Autodesk Fusion 360 part; units mm, degrees
(part 3 of 3)
sketch "Sketch12" plane through (0, 0, 3) normal (0, 0, 1) x (-1, 0, 0)
  circle A0 centre (-5.4, -11) radius 2.5
  circle A1 centre (-5.4, -64) radius 2.5
  line L0 (-15, -66.5) -> (-15, -75)
  line L1 (-15, -75) -> (-2.5, -75)
  arc A2 (-2.5, -75) -> (0, -72.5) centre (-2.5, -72.5) ccw
  line L2 (0, -72.5) -> (0, -60)
  line L3 (0, -60) -> (-8.5, -60)
  arc A3 (-11, -57.5) -> (-8.5, -60) centre (-8.5, -57.5) ccw
  line L4 (-11, -57.5) -> (-11, -17.5)
  arc A4 (-8.5, -15) -> (-11, -17.5) centre (-8.5, -17.5) ccw
  line L5 (-8.5, -15) -> (0, -15)
  line L6 (0, -15) -> (0, -2.5)
  arc A5 (0, -2.5) -> (-2.5, 0) centre (-2.5, -2.5) ccw
  line L7 (-2.5, 0) -> (-57.5, 0)
  arc A6 (-57.5, 0) -> (-60, -2.5) centre (-57.5, -2.5) ccw
  line L8 (-60, -2.5) -> (-60, -25)
  line L9 (-60, -25) -> (-51.5, -25)
  arc A7 (-49, -27.5) -> (-51.5, -25) centre (-51.5, -27.5) ccw
  line L10 (-49, -27.5) -> (-49, -56.5)
  arc A8 (-51.5, -59) -> (-49, -56.5) centre (-51.5, -56.5) ccw
  line L11 (-51.5, -59) -> (-60, -59)
  line L12 (-60, -59) -> (-60, -72.5)
  arc A9 (-60, -72.5) -> (-57.5, -75) centre (-57.5, -72.5) ccw
  line L13 (-57.5, -75) -> (-45, -75)
  line L14 (-45, -75) -> (-45, -66.5)
  arc A10 (-42.5, -64) -> (-45, -66.5) centre (-42.5, -66.5) ccw
  line L15 (-42.5, -64) -> (-17.5, -64)
  arc A11 (-15, -66.5) -> (-17.5, -64) centre (-17.5, -66.5) ccw
  line L16 (-31.117, -41.7434) -> (-30.2084, -42.0729)
  line L17 (-30.2084, -42.0729) -> (-30.2084, -42.4945)
  line L18 (-30.2084, -42.4945) -> (-33.2084, -41.3423)
  line L19 (-33.2084, -41.3423) -> (-33.2084, -40.9146)
  line L20 (-33.2084, -40.9146) -> (-30.2084, -39.6868)
  line L21 (-30.2084, -39.6868) -> (-30.2084, -40.1391)
  line L22 (-30.2084, -40.1391) -> (-31.117, -40.489)
  line L23 (-31.117, -40.489) -> (-31.117, -41.7434)
  line L24 (-32.8544, -35.9604) -> (-30.2084, -35.9604)
  line L25 (-30.2084, -35.9604) -> (-30.2084, -36.3573)
  line L26 (-30.2084, -36.3573) -> (-32.8544, -36.3573)
  line L27 (-32.8544, -36.3573) -> (-32.8544, -37.3458)
  line L28 (-32.8544, -37.3458) -> (-33.2084, -37.3458)
  line L29 (-33.2084, -37.3458) -> (-33.2084, -34.9679)
  line L30 (-33.2084, -34.9679) -> (-32.8544, -34.9679)
  line L31 (-32.8544, -34.9679) -> (-32.8544, -35.9604)
  line L32 (-31.5406, -31.3621) -> (-30.2084, -31.3621)
  line L33 (-30.2084, -31.3621) -> (-30.2084, -31.7591)
  line L34 (-30.2084, -31.7591) -> (-33.2084, -31.7591)
  line L35 (-33.2084, -31.7591) -> (-33.2084, -30.429)
  spline S0 degree 3 poles (-33.2084, -30.429) (-33.2075, -30.3105) (-33.2059, -30.1035) (-33.151, -29.9043) (-33.1276, -29.8192) knots 0 0 0 0 0.035358 0.061746 0.061746 0.061746 0.061746
  spline S1 degree 3 poles (-33.1276, -29.8192) (-33.0949, -29.7527) (-33.0282, -29.6173) (-32.9049, -29.53) (-32.8421, -29.4856) knots 0 0 0 0 0.021851 0.044529 0.044529 0.044529 0.044529
  spline S2 degree 3 poles (-32.8421, -29.4856) (-32.7718, -29.4492) (-32.6298, -29.3757) (-32.4703, -29.3658) (-32.3899, -29.3608) knots 0 0 0 0 0.023485 0.047377 0.047377 0.047377 0.047377
  spline S3 degree 3 poles (-32.3899, -29.3608) (-32.2883, -29.3688) (-32.0883, -29.3846) (-31.9297, -29.5072) (-31.8517, -29.5674) knots 0 0 0 0 0.029867 0.058777 0.058777 0.058777 0.058777
  spline S4 degree 3 poles (-31.8517, -29.5674) (-31.7846, -29.6517) (-31.6358, -29.839) (-31.5955, -30.0758) (-31.5734, -30.2059) knots 0 0 0 0 0.031814 0.070654 0.070654 0.070654 0.070654
  spline S5 degree 3 poles (-31.5734, -30.2059) (-31.55, -30.1586) (-31.5081, -30.0738) (-31.4498, -29.9994) (-31.424, -29.9665) knots 0 0 0 0 0.015773 0.028287 0.028287 0.028287 0.028287
  spline S6 degree 3 poles (-31.424, -29.9665) (-31.3657, -29.9082) (-31.2433, -29.7856) (-31.1, -29.6881) (-31.0249, -29.637) knots 0 0 0 0 0.024682 0.05185 0.05185 0.05185 0.05185
  line L36 (-31.0249, -29.637) -> (-30.2084, -29.1152)
  line L37 (-30.2084, -29.1152) -> (-30.2084, -29.6145)
  line L38 (-30.2084, -29.6145) -> (-30.8326, -30.0115)
  spline S7 degree 3 poles (-30.8326, -30.0115) (-30.9127, -30.0634) (-31.0536, -30.1545) (-31.188, -30.2548) (-31.2459, -30.298) knots 0 0 0 0 0.028634 0.050307 0.050307 0.050307 0.050307
  spline S8 degree 3 poles (-31.2459, -30.298) (-31.2883, -30.3319) (-31.3628, -30.3915) (-31.4212, -30.467) (-31.4465, -30.4996) knots 0 0 0 0 0.016187 0.028522 0.028522 0.028522 0.028522
  spline S9 degree 3 poles (-31.4465, -30.4996) (-31.464, -30.5289) (-31.4981, -30.586) (-31.5171, -30.6497) (-31.5263, -30.6807) knots 0 0 0 0 0.010209 0.01986 0.01986 0.01986 0.01986
  spline S10 degree 3 poles (-31.5263, -30.6807) (-31.5304, -30.7103) (-31.5407, -30.7836) (-31.5406, -30.8576) (-31.5406, -30.9017) knots 0 0 0 0 0.008966 0.02217 0.02217 0.02217 0.02217
  line L39 (-31.5406, -30.9017) -> (-31.5406, -31.3621)
  line L40 (-31.4792, -27.5722) -> (-30.2084, -27.5722)
  line L41 (-30.2084, -27.5722) -> (-30.2084, -27.9692)
  line L42 (-30.2084, -27.9692) -> (-31.4792, -27.9692)
  line L43 (-31.4792, -27.9692) -> (-33.2084, -29.1254)
  line L44 (-33.2084, -29.1254) -> (-33.2084, -28.6425)
  line L45 (-33.2084, -28.6425) -> (-32.3039, -28.0511)
  spline S11 degree 3 poles (-32.3039, -28.0511) (-32.2198, -27.9977) (-32.0531, -27.8919) (-31.8814, -27.7944) (-31.7964, -27.7462) knots 0 0 0 0 0.029896 0.059213 0.059213 0.059213 0.059213
  spline S12 degree 3 poles (-31.7964, -27.7462) (-31.8801, -27.6969) (-32.0592, -27.5916) (-32.2336, -27.4788) (-32.3264, -27.4187) knots 0 0 0 0 0.029138 0.062305 0.062305 0.062305 0.062305
  line L46 (-32.3264, -27.4187) -> (-33.2084, -26.8376)
  line L47 (-33.2084, -26.8376) -> (-33.2084, -26.3751)
  line L48 (-33.2084, -26.3751) -> (-31.4792, -27.5722)
  line L49 (-31.117, -22.178) -> (-30.2084, -22.5074)
  line L50 (-30.2084, -22.5074) -> (-30.2084, -22.929)
  line L51 (-30.2084, -22.929) -> (-33.2084, -21.7769)
  line L52 (-33.2084, -21.7769) -> (-33.2084, -21.3492)
  line L53 (-33.2084, -21.3492) -> (-30.2084, -20.1213)
  line L54 (-30.2084, -20.1213) -> (-30.2084, -20.5736)
  line L55 (-30.2084, -20.5736) -> (-31.117, -20.9235)
  line L56 (-31.117, -20.9235) -> (-31.117, -22.178)
  line L57 (-30.5624, -15.0729) -> (-30.2084, -15.0729)
  line L58 (-30.2084, -15.0729) -> (-30.2084, -17.3116)
  line L59 (-30.2084, -17.3116) -> (-33.2084, -17.3116)
  line L60 (-33.2084, -17.3116) -> (-33.2084, -15.1425)
  line L61 (-33.2084, -15.1425) -> (-32.8544, -15.1425)
  line L62 (-32.8544, -15.1425) -> (-32.8544, -16.9147)
  line L63 (-32.8544, -16.9147) -> (-31.9356, -16.9147)
  line L64 (-31.9356, -16.9147) -> (-31.9356, -15.255)
  line L65 (-31.9356, -15.255) -> (-31.5836, -15.255)
  line L66 (-31.5836, -15.255) -> (-31.5836, -16.9147)
  line L67 (-31.5836, -16.9147) -> (-30.5624, -16.9147)
  line L68 (-30.5624, -16.9147) -> (-30.5624, -15.0729)
  line L69 (-31.4792, -18.873) -> (-30.2084, -18.873)
  line L70 (-30.2084, -18.873) -> (-30.2084, -19.27)
  line L71 (-30.2084, -19.27) -> (-31.4792, -19.27)
  line L72 (-31.4792, -19.27) -> (-33.2084, -20.4262)
  line L73 (-33.2084, -20.4262) -> (-33.2084, -19.9433)
  line L74 (-33.2084, -19.9433) -> (-32.3039, -19.3519)
  spline S13 degree 3 poles (-32.3039, -19.3519) (-32.2198, -19.2985) (-32.0531, -19.1927) (-31.8814, -19.0952) (-31.7964, -19.047) knots 0 0 0 0 0.029897 0.059214 0.059214 0.059214 0.059214
  spline S14 degree 3 poles (-31.7964, -19.047) (-31.8801, -18.9977) (-32.0592, -18.8924) (-32.2336, -18.7796) (-32.3264, -18.7196) knots 0 0 0 0 0.029138 0.062305 0.062305 0.062305 0.062305
  line L75 (-32.3264, -18.7196) -> (-33.2084, -18.1384)
  line L76 (-33.2084, -18.1384) -> (-33.2084, -17.6759)
  line L77 (-33.2084, -17.6759) -> (-31.4792, -18.873)
  line L78 (-30.5624, -23.0722) -> (-30.2084, -23.0722)
  line L79 (-30.2084, -23.0722) -> (-30.2084, -24.9467)
  line L80 (-30.2084, -24.9467) -> (-33.2084, -24.9467)
  line L81 (-33.2084, -24.9467) -> (-33.2084, -24.5497)
  line L82 (-33.2084, -24.5497) -> (-30.5624, -24.5497)
  line L83 (-30.5624, -24.5497) -> (-30.5624, -23.0722)
  line L84 (-31.5406, -14.1213) -> (-30.2084, -14.1213)
  line L85 (-30.2084, -14.1213) -> (-30.2084, -14.5183)
  line L86 (-30.2084, -14.5183) -> (-33.2084, -14.5183)
  line L87 (-33.2084, -14.5183) -> (-33.2084, -13.1882)
  spline S15 degree 3 poles (-33.2084, -13.1882) (-33.2075, -13.0697) (-33.2059, -12.8627) (-33.151, -12.6635) (-33.1276, -12.5784) knots 0 0 0 0 0.035358 0.061746 0.061746 0.061746 0.061746
  spline S16 degree 3 poles (-33.1276, -12.5784) (-33.0949, -12.5119) (-33.0282, -12.3765) (-32.9049, -12.2892) (-32.8421, -12.2448) knots 0 0 0 0 0.021851 0.044528 0.044528 0.044528 0.044528
  spline S17 degree 3 poles (-32.8421, -12.2448) (-32.7718, -12.2084) (-32.6298, -12.1349) (-32.4703, -12.125) (-32.3899, -12.12) knots 0 0 0 0 0.023485 0.047377 0.047377 0.047377 0.047377
  spline S18 degree 3 poles (-32.3899, -12.12) (-32.2883, -12.128) (-32.0883, -12.1438) (-31.9297, -12.2664) (-31.8517, -12.3267) knots 0 0 0 0 0.029867 0.058777 0.058777 0.058777 0.058777
  spline S19 degree 3 poles (-31.8517, -12.3267) (-31.7846, -12.411) (-31.6358, -12.5982) (-31.5955, -12.835) (-31.5734, -12.9651) knots 0 0 0 0 0.031814 0.070654 0.070654 0.070654 0.070654
  spline S20 degree 3 poles (-31.5734, -12.9651) (-31.55, -12.9178) (-31.5081, -12.833) (-31.4498, -12.7586) (-31.424, -12.7257) knots 0 0 0 0 0.015772 0.028287 0.028287 0.028287 0.028287
  spline S21 degree 3 poles (-31.424, -12.7257) (-31.3657, -12.6674) (-31.2433, -12.5448) (-31.1, -12.4473) (-31.0249, -12.3962) knots 0 0 0 0 0.024682 0.05185 0.05185 0.05185 0.05185
  line L88 (-31.0249, -12.3962) -> (-30.2084, -11.8744)
  line L89 (-30.2084, -11.8744) -> (-30.2084, -12.3737)
  line L90 (-30.2084, -12.3737) -> (-30.8326, -12.7707)
  spline S22 degree 3 poles (-30.8326, -12.7707) (-30.9127, -12.8226) (-31.0535, -12.9137) (-31.188, -13.014) (-31.2459, -13.0572) knots 0 0 0 0 0.028634 0.050306 0.050306 0.050306 0.050306
  spline S23 degree 3 poles (-31.2459, -13.0572) (-31.2883, -13.0911) (-31.3628, -13.1507) (-31.4212, -13.2262) (-31.4465, -13.2588) knots 0 0 0 0 0.016188 0.028522 0.028522 0.028522 0.028522
  spline S24 degree 3 poles (-31.4465, -13.2588) (-31.464, -13.2881) (-31.4981, -13.3452) (-31.5171, -13.4089) (-31.5263, -13.4399) knots 0 0 0 0 0.010209 0.01986 0.01986 0.01986 0.01986
  spline S25 degree 3 poles (-31.5263, -13.4399) (-31.5304, -13.4695) (-31.5407, -13.5428) (-31.5406, -13.6168) (-31.5406, -13.6609) knots 0 0 0 0 0.008967 0.02217 0.02217 0.02217 0.02217
  line L91 (-31.5406, -13.6609) -> (-31.5406, -14.1213)
  line L92 (-30.5624, -32.3137) -> (-30.2084, -32.3137)
  line L93 (-30.2084, -32.3137) -> (-30.2084, -34.5524)
  line L94 (-30.2084, -34.5524) -> (-33.2084, -34.5524)
  line L95 (-33.2084, -34.5524) -> (-33.2084, -32.3833)
  line L96 (-33.2084, -32.3833) -> (-32.8544, -32.3833)
  line L97 (-32.8544, -32.3833) -> (-32.8544, -34.1554)
  line L98 (-32.8544, -34.1554) -> (-31.9356, -34.1554)
  line L99 (-31.9356, -34.1554) -> (-31.9356, -32.4958)
  line L100 (-31.9356, -32.4958) -> (-31.5836, -32.4958)
  line L101 (-31.5836, -32.4958) -> (-31.5836, -34.1554)
  line L102 (-31.5836, -34.1554) -> (-30.5624, -34.1554)
  line L103 (-30.5624, -34.1554) -> (-30.5624, -32.3137)
  line L104 (-32.8544, -38.5204) -> (-30.2084, -38.5204)
  line L105 (-30.2084, -38.5204) -> (-30.2084, -38.9174)
  line L106 (-30.2084, -38.9174) -> (-32.8544, -38.9174)
  line L107 (-32.8544, -38.9174) -> (-32.8544, -39.9058)
  line L108 (-32.8544, -39.9058) -> (-33.2084, -39.9058)
  line L109 (-33.2084, -39.9058) -> (-33.2084, -37.5279)
  line L110 (-33.2084, -37.5279) -> (-32.8544, -37.5279)
  line L111 (-32.8544, -37.5279) -> (-32.8544, -38.5204)
  spline S26 degree 3 poles (-30.2586, -43.3488) (-30.244, -43.4218) (-30.212, -43.5815) (-30.2097, -43.7444) (-30.2084, -43.8328) knots 0 0 0 0 0.022292 0.048746 0.048746 0.048746 0.048746
  line L112 (-30.2084, -43.8328) -> (-30.2084, -44.9767)
  line L113 (-30.2084, -44.9767) -> (-33.2084, -44.9767)
  line L114 (-33.2084, -44.9767) -> (-33.2084, -43.8512)
  spline S27 degree 3 poles (-33.2084, -43.8512) (-33.2065, -43.747) (-33.2031, -43.5584) (-33.1438, -43.3796) (-33.1174, -43.2997) knots 0 0 0 0 0.031061 0.05618 0.05618 0.05618 0.05618
  spline S28 degree 3 poles (-33.1174, -43.2997) (-33.0831, -43.2343) (-33.0148, -43.1041) (-32.8961, -43.0175) (-32.837, -42.9743) knots 0 0 0 0 0.021833 0.043463 0.043463 0.043463 0.043463
  spline S29 degree 3 poles (-32.837, -42.9743) (-32.7739, -42.94) (-32.6502, -42.8727) (-32.5098, -42.862) (-32.441, -42.8567) knots 0 0 0 0 0.02128 0.041726 0.041726 0.041726 0.041726
  spline S30 degree 3 poles (-32.441, -42.8567) (-32.3776, -42.8612) (-32.2495, -42.8703) (-32.1361, -42.9306) (-32.0788, -42.961) knots 0 0 0 0 0.018855 0.038069 0.038069 0.038069 0.038069
  spline S31 degree 3 poles (-32.0788, -42.961) (-32.0242, -43.0017) (-31.9101, -43.0867) (-31.8408, -43.2112) (-31.8046, -43.2762) knots 0 0 0 0 0.020176 0.042199 0.042199 0.042199 0.042199
  spline S32 degree 3 poles (-31.8046, -43.2762) (-31.7748, -43.1919) (-31.7176, -43.0302) (-31.5924, -42.9135) (-31.5324, -42.8577) knots 0 0 0 0 0.02638 0.050582 0.050582 0.050582 0.050582
  spline S33 degree 3 poles (-31.5324, -42.8577) (-31.4645, -42.815) (-31.3256, -42.7278) (-31.1618, -42.7169) (-31.0781, -42.7114) knots 0 0 0 0 0.023673 0.048399 0.048399 0.048399 0.048399
  spline S34 degree 3 poles (-31.0781, -42.7114) (-31.0095, -42.7149) (-30.8737, -42.7219) (-30.7482, -42.7744) (-30.6863, -42.8004) knots 0 0 0 0 0.020457 0.040457 0.040457 0.040457 0.040457
  spline S35 degree 3 poles (-30.6863, -42.8004) (-30.6304, -42.8305) (-30.5243, -42.8876) (-30.4446, -42.9778) (-30.4069, -43.0204) knots 0 0 0 0 0.018875 0.035805 0.035805 0.035805 0.035805
  spline S36 degree 3 poles (-30.4069, -43.0204) (-30.3758, -43.0685) (-30.3098, -43.1704) (-30.2763, -43.2872) (-30.2586, -43.3488) knots 0 0 0 0 0.017093 0.036216 0.036216 0.036216 0.036216
  circle A12 centre (-54.6, -16.4) radius 1.4
  circle A13 centre (-5.4, -69.6) radius 1.4
  circle A14 centre (-5.4, -5.4) radius 1.4
  circle A15 centre (-54.6, -69.6) radius 1.4
  spline S37 degree 3 poles (-39.691, -3.4945) (-39.6372, -3.3999) (-39.5038, -3.1654) (-39.5044, -2.8934) (-39.5048, -2.7312) knots 0 0 0 0 0.032195 0.079746 0.079746 0.079746 0.079746
  line L115 (-39.5048, -2.7312) -> (-39.5048, -1)
  line L116 (-39.5048, -1) -> (-39.1078, -1)
  line L117 (-39.1078, -1) -> (-39.1078, -2.7333)
  spline S38 degree 3 poles (-39.1078, -2.7333) (-39.1097, -2.8695) (-39.1131, -3.1137) (-39.1804, -3.348) (-39.2101, -3.4516) knots 0 0 0 0 0.04065 0.072837 0.072837 0.072837 0.072837
  spline S39 degree 3 poles (-39.2101, -3.4516) (-39.2522, -3.5368) (-39.3388, -3.712) (-39.4978, -3.8259) (-39.5795, -3.8844) knots 0 0 0 0 0.028068 0.057686 0.057686 0.057686 0.057686
  spline S40 degree 3 poles (-39.5795, -3.8844) (-39.6807, -3.9329) (-39.9017, -4.039) (-40.1472, -4.0469) (-40.2804, -4.0512) knots 0 0 0 0 0.033312 0.072747 0.072747 0.072747 0.072747
  spline S41 degree 3 poles (-40.2804, -4.0512) (-40.4099, -4.0474) (-40.649, -4.0405) (-40.8692, -3.9482) (-40.97, -3.9059) knots 0 0 0 0 0.03849 0.071015 0.071015 0.071015 0.071015
  spline S42 degree 3 poles (-40.97, -3.9059) (-41.0528, -3.8523) (-41.2175, -3.7458) (-41.3078, -3.5718) (-41.3527, -3.4853) knots 0 0 0 0 0.029047 0.057739 0.057739 0.057739 0.057739
  spline S43 degree 3 poles (-41.3527, -3.4853) (-41.386, -3.3776) (-41.4615, -3.133) (-41.4652, -2.8767) (-41.4673, -2.7333) knots 0 0 0 0 0.033678 0.076416 0.076416 0.076416 0.076416
  line L118 (-41.4673, -2.7333) -> (-41.4673, -1)
  line L119 (-41.4673, -1) -> (-41.0703, -1)
  line L120 (-41.0703, -1) -> (-41.0703, -2.7312)
  spline S44 degree 3 poles (-41.0703, -2.7312) (-41.0699, -2.8452) (-41.0692, -3.0405) (-41.0187, -3.2288) (-40.9976, -3.3073) knots 0 0 0 0 0.033993 0.058274 0.058274 0.058274 0.058274
  spline S45 degree 3 poles (-40.9976, -3.3073) (-40.9689, -3.3656) (-40.911, -3.4829) (-40.8025, -3.556) (-40.748, -3.5928) knots 0 0 0 0 0.01914 0.038515 0.038515 0.038515 0.038515
  spline S46 degree 3 poles (-40.748, -3.5928) (-40.6834, -3.622) (-40.546, -3.6841) (-40.3951, -3.69) (-40.3151, -3.693) knots 0 0 0 0 0.021059 0.044802 0.044802 0.044802 0.044802
  spline S47 degree 3 poles (-40.3151, -3.693) (-40.1854, -3.6901) (-39.9561, -3.685) (-39.7713, -3.5522) (-39.691, -3.4945) knots 0 0 0 0 0.037827 0.066851 0.066851 0.066851 0.066851
  spline S48 degree 3 poles (-34.0399, -3.9499) (-34.1129, -3.9645) (-34.2726, -3.9964) (-34.4355, -3.9987) (-34.5239, -4) knots 0 0 0 0 0.022292 0.048746 0.048746 0.048746 0.048746
  line L121 (-34.5239, -4) -> (-35.6678, -4)
  line L122 (-35.6678, -4) -> (-35.6678, -1)
  line L123 (-35.6678, -1) -> (-34.5423, -1)
  spline S49 degree 3 poles (-34.5423, -1) (-34.438, -1.0019) (-34.2495, -1.0053) (-34.0707, -1.0646) (-33.9908, -1.0911) knots 0 0 0 0 0.031061 0.05618 0.05618 0.05618 0.05618
  spline S50 degree 3 poles (-33.9908, -1.0911) (-33.9254, -1.1254) (-33.7952, -1.1936) (-33.7085, -1.3123) (-33.6654, -1.3714) knots 0 0 0 0 0.021833 0.043463 0.043463 0.043463 0.043463
  spline S51 degree 3 poles (-33.6654, -1.3714) (-33.6311, -1.4345) (-33.5638, -1.5583) (-33.553, -1.6986) (-33.5477, -1.7674) knots 0 0 0 0 0.02128 0.041726 0.041726 0.041726 0.041726
  spline S52 degree 3 poles (-33.5477, -1.7674) (-33.5523, -1.8308) (-33.5614, -1.9589) (-33.6217, -2.0724) (-33.6521, -2.1296) knots 0 0 0 0 0.018855 0.038069 0.038069 0.038069 0.038069
  spline S53 degree 3 poles (-33.6521, -2.1296) (-33.6928, -2.1842) (-33.7778, -2.2983) (-33.9023, -2.3676) (-33.9673, -2.4038) knots 0 0 0 0 0.020176 0.042199 0.042199 0.042199 0.042199
  spline S54 degree 3 poles (-33.9673, -2.4038) (-33.8829, -2.4336) (-33.7213, -2.4908) (-33.6046, -2.6161) (-33.5488, -2.676) knots 0 0 0 0 0.02638 0.050582 0.050582 0.050582 0.050582
  spline S55 degree 3 poles (-33.5488, -2.676) (-33.5061, -2.7439) (-33.4189, -2.8828) (-33.408, -3.0466) (-33.4025, -3.1303) knots 0 0 0 0 0.023673 0.048399 0.048399 0.048399 0.048399
  spline S56 degree 3 poles (-33.4025, -3.1303) (-33.406, -3.199) (-33.413, -3.3348) (-33.4655, -3.4602) (-33.4915, -3.5222) knots 0 0 0 0 0.020457 0.040457 0.040457 0.040457 0.040457
  spline S57 degree 3 poles (-33.4915, -3.5222) (-33.5216, -3.5781) (-33.5787, -3.6841) (-33.6688, -3.7638) (-33.7115, -3.8015) knots 0 0 0 0 0.018874 0.035805 0.035805 0.035805 0.035805
  spline S58 degree 3 poles (-33.7115, -3.8015) (-33.7596, -3.8326) (-33.8615, -3.8986) (-33.9782, -3.9322) (-34.0399, -3.9499) knots 0 0 0 0 0.017093 0.036216 0.036216 0.036216 0.036216
  line L124 (-31.2947, -2.7804) -> (-31.2947, -4)
  line L125 (-31.2947, -4) -> (-31.6917, -4)
  line L126 (-31.6917, -4) -> (-31.6917, -1)
  line L127 (-31.6917, -1) -> (-30.56, -1)
  spline S59 degree 3 poles (-30.56, -1) (-30.4721, -1.0003) (-30.3193, -1.0007) (-30.1679, -1.0203) (-30.1037, -1.0286) knots 0 0 0 0 0.026357 0.045763 0.045763 0.045763 0.045763
  spline S60 degree 3 poles (-30.1037, -1.0286) (-30.0345, -1.0427) (-29.9033, -1.0693) (-29.7879, -1.1369) (-29.7333, -1.1688) knots 0 0 0 0 0.021002 0.039845 0.039845 0.039845 0.039845
  spline S61 degree 3 poles (-29.7333, -1.1688) (-29.6854, -1.2077) (-29.5863, -1.2884) (-29.5247, -1.4004) (-29.4928, -1.4584) knots 0 0 0 0 0.01832 0.037955 0.037955 0.037955 0.037955
  spline S62 degree 3 poles (-29.4928, -1.4584) (-29.4663, -1.5227) (-29.4121, -1.6538) (-29.4053, -1.7955) (-29.4018, -1.8677) knots 0 0 0 0 0.020702 0.042208 0.042208 0.042208 0.042208
  spline S63 degree 3 poles (-29.4018, -1.8677) (-29.4112, -1.9895) (-29.4298, -2.2292) (-29.5743, -2.4211) (-29.6453, -2.5153) knots 0 0 0 0 0.035846 0.070494 0.070494 0.070494 0.070494
  spline S64 degree 3 poles (-29.6453, -2.5153) (-29.7556, -2.5922) (-30.0174, -2.7744) (-30.3391, -2.7782) (-30.5252, -2.7804) knots 0 0 0 0 0.039534 0.09376 0.09376 0.09376 0.09376
  line L128 (-30.5252, -2.7804) -> (-31.2947, -2.7804)
  line L129 (-25.2333, -2.6678) -> (-25.2333, -4)
  line L130 (-25.2333, -4) -> (-25.6303, -4)
  line L131 (-25.6303, -4) -> (-25.6303, -1)
  line L132 (-25.6303, -1) -> (-24.3001, -1)
  spline S65 degree 3 poles (-24.3001, -1) (-24.1816, -1.0009) (-23.9747, -1.0025) (-23.7754, -1.0574) (-23.6903, -1.0808) knots 0 0 0 0 0.035358 0.061746 0.061746 0.061746 0.061746
  spline S66 degree 3 poles (-23.6903, -1.0808) (-23.6239, -1.1135) (-23.4884, -1.1802) (-23.4012, -1.3035) (-23.3568, -1.3663) knots 0 0 0 0 0.021851 0.044529 0.044529 0.044529 0.044529
  spline S67 degree 3 poles (-23.3568, -1.3663) (-23.3203, -1.4367) (-23.2469, -1.5786) (-23.2369, -1.7381) (-23.2319, -1.8186) knots 0 0 0 0 0.023485 0.047377 0.047377 0.047377 0.047377
  spline S68 degree 3 poles (-23.2319, -1.8186) (-23.24, -1.9202) (-23.2558, -2.1202) (-23.3783, -2.2787) (-23.4386, -2.3568) knots 0 0 0 0 0.029867 0.058777 0.058777 0.058777 0.058777
  spline S69 degree 3 poles (-23.4386, -2.3568) (-23.5229, -2.4238) (-23.7101, -2.5726) (-23.9469, -2.6129) (-24.0771, -2.6351) knots 0 0 0 0 0.031814 0.070654 0.070654 0.070654 0.070654
  spline S70 degree 3 poles (-24.0771, -2.6351) (-24.0298, -2.6584) (-23.945, -2.7003) (-23.8706, -2.7587) (-23.8377, -2.7844) knots 0 0 0 0 0.015773 0.028287 0.028287 0.028287 0.028287
  spline S71 degree 3 poles (-23.8377, -2.7844) (-23.7793, -2.8427) (-23.6568, -2.9652) (-23.5593, -3.1084) (-23.5082, -3.1835) knots 0 0 0 0 0.024682 0.05185 0.05185 0.05185 0.05185
  line L133 (-23.5082, -3.1835) -> (-22.9864, -4)
  line L134 (-22.9864, -4) -> (-23.4857, -4)
  line L135 (-23.4857, -4) -> (-23.8827, -3.3759)
  spline S72 degree 3 poles (-23.8827, -3.3759) (-23.9346, -3.2957) (-24.0257, -3.1549) (-24.126, -3.0204) (-24.1692, -2.9625) knots 0 0 0 0 0.028634 0.050307 0.050307 0.050307 0.050307
  spline S73 degree 3 poles (-24.1692, -2.9625) (-24.203, -2.9202) (-24.2627, -2.8456) (-24.3381, -2.7872) (-24.3707, -2.7619) knots 0 0 0 0 0.016188 0.028522 0.028522 0.028522 0.028522
  spline S74 degree 3 poles (-24.3707, -2.7619) (-24.4001, -2.7444) (-24.4572, -2.7103) (-24.5209, -2.6913) (-24.5518, -2.6821) knots 0 0 0 0 0.01021 0.01986 0.01986 0.01986 0.01986
  spline S75 degree 3 poles (-24.5518, -2.6821) (-24.5815, -2.678) (-24.6547, -2.6677) (-24.7288, -2.6678) (-24.7728, -2.6678) knots 0 0 0 0 0.008966 0.02217 0.02217 0.02217 0.02217
  line L136 (-24.7728, -2.6678) -> (-25.2333, -2.6678)
  spline S76 degree 3 poles (-28.3397, -3.8465) (-28.4442, -3.772) (-28.6535, -3.6227) (-28.7812, -3.3996) (-28.8452, -3.2879) knots 0 0 0 0 0.038012 0.076138 0.076138 0.076138 0.076138
  spline S77 degree 3 poles (-28.8452, -3.2879) (-28.8953, -3.1681) (-28.9957, -2.9283) (-29.0099, -2.6688) (-29.0171, -2.5389) knots 0 0 0 0 0.03864 0.077351 0.077351 0.077351 0.077351
  spline S78 degree 3 poles (-29.0171, -2.5389) (-29.0054, -2.3091) (-28.9837, -1.8792) (-28.7328, -1.5313) (-28.616, -1.3694) knots 0 0 0 0 0.067335 0.126001 0.126001 0.126001 0.126001
  spline S79 degree 3 poles (-28.616, -1.3694) (-28.4701, -1.2461) (-28.1712, -0.9936) (-27.7805, -0.9626) (-27.5805, -0.9468) knots 0 0 0 0 0.055813 0.114379 0.114379 0.114379 0.114379
  spline S80 degree 3 poles (-27.5805, -0.9468) (-27.4465, -0.9545) (-27.1831, -0.9695) (-26.9473, -1.0874) (-26.8315, -1.1453) knots 0 0 0 0 0.039806 0.078211 0.078211 0.078211 0.078211
  spline S81 degree 3 poles (-26.8315, -1.1453) (-26.7268, -1.2183) (-26.5162, -1.365) (-26.3876, -1.5872) (-26.323, -1.6988) knots 0 0 0 0 0.037796 0.075988 0.075988 0.075988 0.075988
  spline S82 degree 3 poles (-26.323, -1.6988) (-26.272, -1.8235) (-26.1664, -2.0815) (-26.1543, -2.3601) (-26.148, -2.5041) knots 0 0 0 0 0.040092 0.082957 0.082957 0.082957 0.082957
  spline S83 degree 3 poles (-26.148, -2.5041) (-26.1547, -2.6502) (-26.1676, -2.9335) (-26.2785, -3.1943) (-26.3322, -3.3206) knots 0 0 0 0 0.043474 0.084303 0.084303 0.084303 0.084303
  spline S84 degree 3 poles (-26.3322, -3.3206) (-26.3992, -3.4329) (-26.5315, -3.6547) (-26.7475, -3.7962) (-26.854, -3.866) knots 0 0 0 0 0.038684 0.076365 0.076365 0.076365 0.076365
  spline S85 degree 3 poles (-26.854, -3.866) (-26.969, -3.92) (-27.2, -4.0284) (-27.4547, -4.0436) (-27.5825, -4.0512) knots 0 0 0 0 0.037744 0.075783 0.075783 0.075783 0.075783
  spline S86 degree 3 poles (-27.5825, -4.0512) (-27.7188, -4.0434) (-27.9856, -4.0281) (-28.2233, -3.9062) (-28.3397, -3.8465) knots 0 0 0 0 0.040434 0.079208 0.079208 0.079208 0.079208
  line L137 (-21.5252, -1.354) -> (-21.5252, -4)
  line L138 (-21.5252, -4) -> (-21.9222, -4)
  line L139 (-21.9222, -4) -> (-21.9222, -1.354)
  line L140 (-21.9222, -1.354) -> (-22.9106, -1.354)
  line L141 (-22.9106, -1.354) -> (-22.9106, -1)
  line L142 (-22.9106, -1) -> (-20.5327, -1)
  line L143 (-20.5327, -1) -> (-20.5327, -1.354)
  line L144 (-20.5327, -1.354) -> (-21.5252, -1.354)
  spline S87 degree 3 poles (-37.9853, -3.9325) (-38.0718, -3.8885) (-38.2424, -3.8016) (-38.3594, -3.6501) (-38.4171, -3.5754) knots 0 0 0 0 0.028704 0.056657 0.056657 0.056657 0.056657
  spline S88 degree 3 poles (-38.4171, -3.5754) (-38.4631, -3.4926) (-38.5565, -3.3247) (-38.5733, -3.1332) (-38.5819, -3.0362) knots 0 0 0 0 0.02807 0.056948 0.056948 0.056948 0.056948
  line L145 (-38.5819, -3.0362) -> (-38.2074, -3.0034)
  spline S89 degree 3 poles (-38.2074, -3.0034) (-38.1968, -3.0732) (-38.177, -3.2037) (-38.1133, -3.3191) (-38.0836, -3.3728) knots 0 0 0 0 0.020962 0.039233 0.039233 0.039233 0.039233
  spline S90 degree 3 poles (-38.0836, -3.3728) (-38.0447, -3.4194) (-37.9614, -3.5192) (-37.8442, -3.5759) (-37.7817, -3.6061) knots 0 0 0 0 0.018003 0.038541 0.038541 0.038541 0.038541
  spline S91 degree 3 poles (-37.7817, -3.6061) (-37.71, -3.632) (-37.5612, -3.6858) (-37.4031, -3.6919) (-37.3213, -3.6951) knots 0 0 0 0 0.022745 0.047147 0.047147 0.047147 0.047147
  spline S92 degree 3 poles (-37.3213, -3.6951) (-37.2494, -3.6929) (-37.1125, -3.6887) (-36.9821, -3.6472) (-36.9202, -3.6276) knots 0 0 0 0 0.021451 0.040849 0.040849 0.040849 0.040849
  spline S93 degree 3 poles (-36.9202, -3.6276) (-36.867, -3.6044) (-36.7673, -3.5611) (-36.6951, -3.4801) (-36.6613, -3.4424) knots 0 0 0 0 0.017152 0.032166 0.032166 0.032166 0.032166
  spline S94 degree 3 poles (-36.6613, -3.4424) (-36.6366, -3.4025) (-36.5876, -3.3237) (-36.5801, -3.2312) (-36.5764, -3.1855) knots 0 0 0 0 0.013855 0.0274 0.0274 0.0274 0.0274
  spline S95 degree 3 poles (-36.5764, -3.1855) (-36.5796, -3.1402) (-36.5859, -3.051) (-36.6344, -2.9759) (-36.6583, -2.9389) knots 0 0 0 0 0.013382 0.02636 0.02636 0.02636 0.02636
  spline S96 degree 3 poles (-36.6583, -2.9389) (-36.6928, -2.9042) (-36.7701, -2.8264) (-36.872, -2.7849) (-36.9284, -2.7619) knots 0 0 0 0 0.014547 0.032588 0.032588 0.032588 0.032588
  spline S97 degree 3 poles (-36.9284, -2.7619) (-36.9928, -2.7413) (-37.1687, -2.6849) (-37.3486, -2.6425) (-37.4625, -2.6156) knots 0 0 0 0 0.0203 0.055396 0.055396 0.055396 0.055396
  spline S98 degree 3 poles (-37.4625, -2.6156) (-37.5809, -2.5873) (-37.779, -2.54) (-37.9663, -2.4604) (-38.0416, -2.4284) knots 0 0 0 0 0.036446 0.060956 0.060956 0.060956 0.060956
  spline S99 degree 3 poles (-38.0416, -2.4284) (-38.1076, -2.3903) (-38.2327, -2.318) (-38.3204, -2.2033) (-38.3619, -2.149) knots 0 0 0 0 0.022596 0.04287 0.04287 0.04287 0.04287
  spline S100 degree 3 poles (-38.3619, -2.149) (-38.3926, -2.0914) (-38.4548, -1.9746) (-38.4631, -1.8425) (-38.4673, -1.7756) knots 0 0 0 0 0.019362 0.039209 0.039209 0.039209 0.039209
  spline S101 degree 3 poles (-38.4673, -1.7756) (-38.4617, -1.7008) (-38.4504, -1.5497) (-38.3759, -1.4176) (-38.3383, -1.351) knots 0 0 0 0 0.022208 0.044864 0.044864 0.044864 0.044864
  spline S102 degree 3 poles (-38.3383, -1.351) (-38.2891, -1.2886) (-38.1871, -1.1594) (-38.0386, -1.088) (-37.9618, -1.0512) knots 0 0 0 0 0.02352 0.0487 0.0487 0.0487 0.0487
  spline S103 degree 3 poles (-37.9618, -1.0512) (-37.8755, -1.0213) (-37.6972, -0.9597) (-37.5086, -0.9525) (-37.4113, -0.9488) knots 0 0 0 0 0.027246 0.056264 0.056264 0.056264 0.056264
  spline S104 degree 3 poles (-37.4113, -0.9488) (-37.3057, -0.9524) (-37.1041, -0.9592) (-36.9136, -1.025) (-36.823, -1.0563) knots 0 0 0 0 0.031501 0.060107 0.060107 0.060107 0.060107
  spline S105 degree 3 poles (-36.823, -1.0563) (-36.7436, -1.0953) (-36.5891, -1.1713) (-36.4828, -1.3066) (-36.4311, -1.3724) knots 0 0 0 0 0.026156 0.050928 0.050928 0.050928 0.050928
  spline S106 degree 3 poles (-36.4311, -1.3724) (-36.3907, -1.445) (-36.3086, -1.5922) (-36.2921, -1.76) (-36.2838, -1.8452) knots 0 0 0 0 0.024624 0.04999 0.04999 0.04999 0.04999
  line L146 (-36.2838, -1.8452) -> (-36.6644, -1.8738)
  spline S107 degree 3 poles (-36.6644, -1.8738) (-36.6787, -1.7865) (-36.7056, -1.6222) (-36.819, -1.5009) (-36.8721, -1.4441) knots 0 0 0 0 0.025856 0.048693 0.048693 0.048693 0.048693
  spline S108 degree 3 poles (-36.8721, -1.4441) (-36.9434, -1.4018) (-37.1038, -1.3068) (-37.291, -1.3016) (-37.395, -1.2988) knots 0 0 0 0 0.024481 0.055061 0.055061 0.055061 0.055061
  spline S109 degree 3 poles (-37.395, -1.2988) (-37.5013, -1.3004) (-37.6877, -1.3032) (-37.8501, -1.3925) (-37.9198, -1.4308) knots 0 0 0 0 0.031305 0.054847 0.054847 0.054847 0.054847
  spline S110 degree 3 poles (-37.9198, -1.4308) (-37.9679, -1.4758) (-38.0606, -1.5627) (-38.0768, -1.6884) (-38.0846, -1.749) knots 0 0 0 0 0.019092 0.036842 0.036842 0.036842 0.036842
  spline S111 degree 3 poles (-38.0846, -1.749) (-38.0799, -1.8003) (-38.0706, -1.902) (-38.002, -1.9776) (-37.9679, -2.015) knots 0 0 0 0 0.01502 0.029764 0.029764 0.029764 0.029764
  spline S112 degree 3 poles (-37.9679, -2.015) (-37.9, -2.0529) (-37.7132, -2.157) (-37.5031, -2.2009) (-37.3694, -2.2289) knots 0 0 0 0 0.023235 0.063865 0.063865 0.063865 0.063865
  spline S113 degree 3 poles (-37.3694, -2.2289) (-37.2323, -2.2595) (-37.0069, -2.3098) (-36.7902, -2.3891) (-36.7053, -2.4202) knots 0 0 0 0 0.042069 0.06917 0.06917 0.06917 0.06917
  spline S114 degree 3 poles (-36.7053, -2.4202) (-36.6254, -2.4608) (-36.4756, -2.5368) (-36.3685, -2.6659) (-36.3186, -2.7261) knots 0 0 0 0 0.026563 0.04978 0.04978 0.04978 0.04978
  spline S115 degree 3 poles (-36.3186, -2.7261) (-36.2821, -2.791) (-36.2078, -2.9235) (-36.1985, -3.0753) (-36.1937, -3.1528) knots 0 0 0 0 0.022016 0.04497 0.04497 0.04497 0.04497
  spline S116 degree 3 poles (-36.1937, -3.1528) (-36.1997, -3.2319) (-36.212, -3.3924) (-36.2908, -3.5328) (-36.3308, -3.604) knots 0 0 0 0 0.023503 0.047671 0.047671 0.047671 0.047671
  spline S117 degree 3 poles (-36.3308, -3.604) (-36.3827, -3.6712) (-36.4898, -3.8099) (-36.6449, -3.8915) (-36.7248, -3.9335) knots 0 0 0 0 0.025169 0.051893 0.051893 0.051893 0.051893
  spline S118 degree 3 poles (-36.7248, -3.9335) (-36.8147, -3.9678) (-37.0008, -4.0388) (-37.2, -4.0469) (-37.3029, -4.0512) knots 0 0 0 0 0.028685 0.059343 0.059343 0.059343 0.059343
  spline S119 degree 3 poles (-37.3029, -4.0512) (-37.4288, -4.048) (-37.6624, -4.042) (-37.8835, -3.967) (-37.9853, -3.9325) knots 0 0 0 0 0.037541 0.069624 0.069624 0.069624 0.069624
  circle A16 centre (-54.6, -64) radius 2.5
  circle A17 centre (-54.6, -22) radius 2.5
  circle A18 centre (-5.4, -69.6) radius 2.75
  circle A19 centre (-54.6, -69.6) radius 2.75
  circle A20 centre (-54.6, -16.4) radius 2.75
  circle A21 centre (-5.4, -5.4) radius 2.75
  dimension "d89" = 5.5
  dimension "d90" = 5.5
  dimension "d91" = 5.5
  dimension "d92" = 5.5
  constraint concentric A13 A18
  constraint concentric A15 A19
  constraint concentric A12 A20
  constraint concentric A14 A21
  measures "d89" diameter of A18
  measures "d90" diameter of A19
  measures "d91" diameter of A20
  measures "d92" diameter of A21
extrude "Extrude13" cut sketch "Sketch12" against normal blind 1.5 contours A18
extrude "Extrude14" cut sketch "Sketch12" against normal blind 1.5 contours A19 | A20 | A21
sketch "Sketch13" plane through (0, 0, 0) normal (0, 0, -1) x (1, 0, 0)
  circle A0 centre (54.6, -69.6) radius 1.4
  circle A1 centre (5.4, -5.4) radius 1.4
  circle A2 centre (5.4, -69.6) radius 1.4
  circle A3 centre (54.6, -16.4) radius 1.4
  line L0 (15, -75) -> (15, -66.5)
  arc A4 (17.5, -64) -> (15, -66.5) centre (17.5, -66.5) ccw
  line L1 (17.5, -64) -> (42.5, -64)
  arc A5 (45, -66.5) -> (42.5, -64) centre (42.5, -66.5) ccw
  line L2 (45, -66.5) -> (45, -75)
  line L3 (45, -75) -> (57.5, -75)
  arc A6 (57.5, -75) -> (60, -72.5) centre (57.5, -72.5) ccw
  line L4 (60, -72.5) -> (60, -59)
  line L5 (60, -59) -> (51.5, -59)
  arc A7 (49, -56.5) -> (51.5, -59) centre (51.5, -56.5) ccw
  line L6 (49, -56.5) -> (49, -27.5)
  arc A8 (51.5, -25) -> (49, -27.5) centre (51.5, -27.5) ccw
  line L7 (51.5, -25) -> (60, -25)
  line L8 (60, -25) -> (60, -2.5)
  arc A9 (60, -2.5) -> (57.5, 0) centre (57.5, -2.5) ccw
  line L9 (57.5, 0) -> (2.5, 0)
  arc A10 (2.5, 0) -> (0, -2.5) centre (2.5, -2.5) ccw
  line L10 (0, -2.5) -> (0, -15)
  line L11 (0, -15) -> (8.5, -15)
  arc A11 (11, -17.5) -> (8.5, -15) centre (8.5, -17.5) ccw
  line L12 (11, -17.5) -> (11, -57.5)
  arc A12 (8.5, -60) -> (11, -57.5) centre (8.5, -57.5) ccw
  line L13 (8.5, -60) -> (0, -60)
  line L14 (0, -60) -> (0, -72.5)
  arc A13 (0, -72.5) -> (2.5, -75) centre (2.5, -72.5) ccw
  line L15 (2.5, -75) -> (15, -75)
  circle A14 centre (5.4, -11) radius 1.4
  circle A15 centre (54.6, -64) radius 1.4
  circle A16 centre (54.6, -22) radius 1.4
  circle A17 centre (5.4, -64) radius 1.4
  line L16 (56.0874, -24.8707) -> (57.8298, -22.1473)
  line L17 (57.8298, -22.1473) -> (56.3424, -19.2765)
  line L18 (56.3424, -19.2765) -> (53.1126, -19.1293)
  line L19 (53.1126, -19.1293) -> (51.3702, -21.8527)
  line L20 (51.3702, -21.8527) -> (52.8576, -24.7235)
  line L21 (52.8576, -24.7235) -> (56.0874, -24.8707)
  line L22 (52.1049, -61.9438) -> (51.5718, -65.1327)
  line L23 (51.5718, -65.1327) -> (54.0669, -67.1889)
  line L24 (54.0669, -67.1889) -> (57.0951, -66.0562)
  line L25 (57.0951, -66.0562) -> (57.6282, -62.8673)
  line L26 (57.6282, -62.8673) -> (55.1331, -60.8111)
  line L27 (55.1331, -60.8111) -> (52.1049, -61.9438)
  line L28 (7.2988, -61.3832) -> (4.0832, -61.0472)
  line L29 (4.0832, -61.0472) -> (2.1843, -63.664)
  line L30 (2.1843, -63.664) -> (3.5012, -66.6168)
  line L31 (3.5012, -66.6168) -> (6.7168, -66.9528)
  line L32 (6.7168, -66.9528) -> (8.6157, -64.336)
  line L33 (8.6157, -64.336) -> (7.2988, -61.3832)
  line L34 (8.2, -9.3834) -> (5.4, -7.7668)
  line L35 (5.4, -7.7668) -> (2.6, -9.3834)
  line L36 (2.6, -9.3834) -> (2.6, -12.6166)
  line L37 (2.6, -12.6166) -> (5.4, -14.2332)
  line L38 (5.4, -14.2332) -> (8.2, -12.6166)
  line L39 (8.2, -12.6166) -> (8.2, -9.3834)
  point P0 (54.6, -22)
  point P1 (54.6, -64)
  point P2 (5.4, -64)
  point P3 (5.4, -11)
  dimension "d97" = 2.8
  dimension "d98" = 2.8
  dimension "d99" = 2.8
  dimension "d100" = 2.8
  constraint coincident P0 A16.centre
  constraint coincident P1 A15.centre
  constraint coincident P2 A17.centre
  constraint coincident P3 A14.centre
  measures "d97" distance of P0 L21
  measures "d98" distance of P1 L27
  measures "d99" distance of P2 L33
  measures "d100" distance of P3 L39
extrude "Extrude15" cut sketch "Sketch13" against normal blind 1.5 contours L16 L17 L18 L19 L20 L21 | L22 L23 L24 L25 L26 L27 | L28 L29 L30 L31 L32 L33 | L34 L35 L36 L37 L38 L39
equation "d22 = 'USB PORT'"
equation "d31 = 'BATTERY LAYER '"
